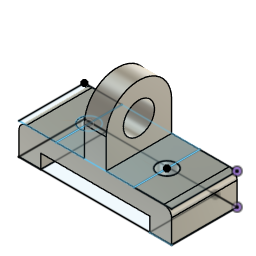
3dShape2 (Autodesk Fusion 360 design; units mm, degrees)
Autodesk Fusion 360 part; units mm, degrees
note: some values were not read from the file. Set by a fixed rule: which sketch regions a step uses.
sketch "Sketch1" plane through (0, 0, 0) normal (0, 0, 1) x (1, 0, 0)
  line L0 (0, 0) -> (-98, 0)
  line L1 (-98, 0) -> (-98, -42)
  line L2 (-98, -42) -> (0, -42)
  line L3 (0, -42) -> (0, 0)
  line L4 (0, 0) -> (-14, 0)
  line L5 (0, 0) -> (-14, 0)
  line L6 (-14, 0) -> (-14, -42)
  line L7 (-14, -42) -> (0, -42)
  line L8 (0, -42) -> (0, 0)
  line L9 (-98, 0) -> (-84, 0)
  line L10 (-98, 0) -> (-98, -42)
  line L11 (-84, 0) -> (-98, 0)
  line L12 (-98, 0) -> (-98, -42)
  line L13 (-98, -42) -> (-84, -42)
  line L14 (-84, -42) -> (-84, 0)
  dimension "d1" = 98
  dimension "d2" = 42
  dimension "d3" = 14
  dimension "d4" = 14
  dimension "d5" = 14
  constraint horizontal L0
  constraint vertical L1
  constraint horizontal L2
  constraint vertical L3
  constraint coincident L0.start L3.end
  constraint perpendicular L3 L4
  constraint horizontal L5
  constraint vertical L6
  constraint horizontal L7
  constraint vertical L8
  constraint perpendicular L1 L9
  constraint horizontal L11
  constraint vertical L12
  constraint horizontal L13
  constraint vertical L14
  measures "d1" distance of L0.start L0.end
  measures "d2" distance of L0.start L2.end
  measures "d3" distance of L0.start L4.end
  measures "d4" distance of L0.start L4.end
  measures "d5" distance of L0.end L9.end
extrude "Extrude1" add sketch "Sketch1" along normal blind 20
extrude "Extrude2" cut sketch "Sketch1" along normal blind 9 contours L0 L2 L6 L14
sketch "Sketch2" plane through (0, 0, 0) normal (0, 0, 1) x (1, 0, 0)
sketch "Sketch3" plane through (0, 0, 20) normal (0, 0, 1) x (-1, 0, 0)
  line L0 (98, 42) -> (0, 42)
  line L1 (0, 42) -> (0, 0)
  line L2 (0, 0) -> (98, 0)
  line L3 (98, 0) -> (98, 42)
  line L4 (0, 0) -> (24, 0)
  line L5 (24, 0) -> (24, 42)
  line L6 (24, 42) -> (0, 42)
  line L7 (0, 42) -> (0, 0)
  circle A0 centre (24, 21) radius 6
  line L8 (98, 0) -> (74, 0)
  line L9 (74, 0) -> (74, 42)
  line L10 (74, 42) -> (98, 42)
  line L11 (98, 42) -> (98, 0)
  circle A1 centre (74, 21) radius 6
  dimension "d10" = 24
  dimension "d11" = 42
  dimension "d12" = 12
  dimension "d13" = 24
  dimension "d14" = 12
  constraint horizontal L4
  constraint vertical L5
  constraint horizontal L6
  constraint vertical L7
  constraint coincident L1.end L2.start
  constraint midpoint L5 A0.centre
  constraint horizontal L8
  constraint vertical L9
  constraint horizontal L10
  constraint vertical L11
  constraint coincident L2.end L3.start
  constraint midpoint L9 A1.centre
  measures "d10" distance of L1.end L4.end
  measures "d11" distance of L1.end L0.end
  measures "d12" diameter of A0
  measures "d13" distance of L2.end L8.end
  measures "d14" diameter of A1
extrude "Extrude3" cut sketch "Sketch3" against normal blind 15 contours L5 A0 | L5 A0
extrude "Extrude4" cut sketch "Sketch3" against normal blind 15 contours L9 A1 | L9 A1
sketch "Sketch4" plane through (0, 0, 20) normal (0, 0, 1) x (-1, 0, 0)
  line L0 (74, 0) -> (24, 0)
  line L1 (24, 0) -> (24, 42)
  line L2 (24, 42) -> (74, 42)
  line L3 (74, 42) -> (74, 0)
  constraint horizontal L0
  constraint vertical L1
  constraint horizontal L2
  constraint vertical L3
extrude "Extrude5" add sketch "Sketch3" along normal blind 40 contours L0 L2 L5 A0 L9 A1
sketch "Sketch5" plane through (0, 0, 60) normal (0, 0, 1) x (-1, 0, 0)
  line L0 (24, 0) -> (74, 0)
  line L1 (74, 0) -> (74, 15)
  arc A0 (74, 27) -> (74, 15) centre (74, 21) ccw
  line L2 (74, 27) -> (74, 42)
  line L3 (74, 42) -> (24, 42)
  line L4 (24, 42) -> (24, 27)
  arc A1 (24, 15) -> (24, 27) centre (24, 21) ccw
  line L5 (24, 15) -> (24, 0)
  line L6 (74, 0) -> (24, 0)
  line L7 (24, 0) -> (24, 42)
  line L8 (24, 42) -> (74, 42)
  line L9 (74, 42) -> (74, 0)
  line L10 (74, 0) -> (49, 0)
  line L11 (74, 0) -> (49, 0)
  line L12 (49, 0) -> (49, 42)
  line L13 (49, 42) -> (74, 42)
  line L14 (74, 42) -> (74, 0)
  line L15 (49, 0) -> (42, 0)
  line L16 (42, 0) -> (42, 42)
  line L17 (42, 42) -> (49, 42)
  line L18 (49, 42) -> (49, 0)
  line L19 (49, 0) -> (56, 0)
  line L20 (56, 0) -> (56, 42)
  line L21 (56, 42) -> (49, 42)
  line L22 (49, 42) -> (49, 0)
  dimension "d21" = 25
  dimension "d22" = 7
  dimension "d23" = 7
  constraint horizontal L6
  constraint vertical L7
  constraint horizontal L8
  constraint vertical L9
  constraint coincident L3.end L4.start
  constraint coincident L0.end L1.start
  constraint midpoint L6 L10.end
  constraint horizontal L11
  constraint vertical L12
  constraint horizontal L13
  constraint vertical L14
  constraint horizontal L15
  constraint vertical L16
  constraint horizontal L17
  constraint vertical L18
  constraint horizontal L19
  constraint vertical L20
  constraint horizontal L21
  constraint vertical L22
  measures "d21" distance of L0.end L10.end
  measures "d22" distance of L10.end L15.end
  measures "d23" distance of L10.end L19.end
extrude "Extrude6" cut sketch "Sketch5" against normal blind 40 contours L0 L1 A0 L2 L3 L6 L8 L9 L10 L11 L13 L14 L20
extrude "Extrude7" cut sketch "Sketch5" against normal blind 40 contours L0 L3 L4 A1 L5 L6 L7 L8 L16
sketch "Sketch6" plane through (0, 0, 60) normal (0, 0, 1) x (-1, 0, 0)
fillet "Fillet1" radius 5 1 edges at (-98, -21, 20)
fillet "Fillet2" radius 5 1 edges at (0, -21, 20)
fillet "Fillet3" radius 21 1 edges at (-49, 0, 60)
fillet "Fillet4" radius 21 1 edges at (-49, -42, 60)
sketch "Sketch7" plane through (-42, 0, 0) normal (1, 0, 0) x (0, 1, 0)
  arc A0 (0, 39) -> (-42, 39) centre (-21, 39) ccw
  line L0 (-42, 39) -> (-42, 20)
  line L1 (-42, 20) -> (0, 20)
  line L2 (0, 20) -> (0, 39)
  line L3 (-42, 39) -> (0, 39)
  line L4 (0, 39) -> (0, 20)
  line L5 (0, 20) -> (-42, 20)
  line L6 (-42, 20) -> (-42, 39)
  circle A1 centre (-21, 39) radius 10
  dimension "d36" = 20
  constraint horizontal L3
  constraint vertical L4
  constraint horizontal L5
  constraint vertical L6
  constraint coincident L1.end L2.start
  constraint coincident A0.end L0.start
  constraint concentric A0 A1
  measures "d36" diameter of A1
extrude "Extrude8" cut sketch "Sketch7" against normal blind 14 contours L3 A1 | L3 A1
